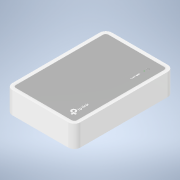
# Autodesk Inventor part: Network Switch (TL-SF1005D)
Saved by Autodesk Inventor 2020.1 (Build 241239000, 239)
## iProperties
Created: 2020-02-09
Part Number: Network Switch (TL-SF1005D)
Material: Generic
Document SubType Name: Modeling
Designer: tejas
Density: 1 g/cm^3
Appearance: Smooth - White
Author: tejas
Autodesk Inventor part; units mm, degrees
(part 1 of 2)
ref_plane "YZ Plane" through (0, 0, 0) normal (1, 0, 0) x (0, 1, 0)
ref_plane "XZ Plane" through (0, 0, 0) normal (0, 1, 0) x (-1, 0, 0)
ref_plane "XY Plane" through (0, 0, 0) normal (0, 0, 1) x (1, 0, 0)
sketch "Sketch1" plane through (0, 0, 0) normal (0, 1, 0) x (-1, 0, 0)
  line L0 (0, 0) -> (-71.12, 0)
  line L1 (-71.12, 0) -> (-71.12, -104.14)
  line L2 (-71.12, -104.14) -> (0, -104.14)
  line L3 (0, -104.14) -> (0, 0)
  dimension "d0" = 71.12
  dimension "d1" = 104.14
  constraints: 8 end point, 2 parallel, 1 horizontal, 1 perpendicular
  measures "d0" distance of L2.end L1.end
  measures "d1" distance of L1.end L0.end
extrude "Extrusion1" add sketch "Sketch1" along normal blind 22.86
sketch "Sketch2" plane through (0, 0, -104.14) normal (-1, 0, 0) x (0, 0, 1)
  line L0 (28.8163, 10.485) -> (16.9037, 10.485)
  line L1 (16.9037, 10.485) -> (16.9037, 12.4916)
  line L2 (16.9037, 12.4916) -> (16.51, 12.4916)
  line L3 (16.51, 12.4916) -> (16.51, 15.2856)
  line L4 (16.51, 15.2856) -> (16.9037, 15.2856)
  line L5 (16.9037, 15.2856) -> (16.9037, 17.3176)
  line L6 (16.9037, 17.3176) -> (19.7104, 17.3176)
  line L7 (19.7104, 17.3176) -> (19.7104, 18.222)
  line L8 (19.7104, 18.222) -> (20.828, 18.222)
  line L9 (20.828, 18.222) -> (20.828, 19.365)
  line L10 (20.828, 19.365) -> (24.892, 19.365)
  line L11 (22.86, 19.365) -> (22.86, 10.485) construction
  line L12 (28.8163, 10.485) -> (28.8163, 12.4916)
  line L13 (28.8163, 12.4916) -> (29.21, 12.4916)
  line L14 (29.21, 12.4916) -> (29.21, 15.2856)
  line L15 (29.21, 15.2856) -> (28.8163, 15.2856)
  line L16 (28.8163, 15.2856) -> (28.8163, 17.3176)
  line L17 (28.8163, 17.3176) -> (26.0096, 17.3176)
  line L18 (26.0096, 17.3176) -> (26.0096, 18.222)
  line L19 (26.0096, 18.222) -> (24.892, 18.222)
  line L20 (24.892, 18.222) -> (24.892, 19.365)
  line L21 (29.21, 13.8886) -> (30.48, 13.8886) construction
  line L22 (30.48, 13.8886) -> (30.48, 20.2386) construction
  line L23 (32.1437, 10.485) -> (44.0563, 10.485)
  line L24 (44.0563, 10.485) -> (44.0563, 12.4916)
  line L25 (44.0563, 12.4916) -> (44.45, 12.4916)
  line L26 (44.45, 12.4916) -> (44.45, 15.2856)
  line L27 (44.45, 15.2856) -> (44.0563, 15.2856)
  line L28 (44.0563, 15.2856) -> (44.0563, 17.3176)
  line L29 (44.0563, 17.3176) -> (41.2496, 17.3176)
  line L30 (41.2496, 17.3176) -> (41.2496, 18.222)
  line L31 (41.2496, 18.222) -> (40.132, 18.222)
  line L32 (40.132, 18.222) -> (40.132, 19.365)
  line L33 (40.132, 19.365) -> (36.068, 19.365)
  line L34 (38.1, 19.365) -> (38.1, 10.485) construction
  line L35 (36.068, 18.222) -> (36.068, 19.365)
  line L36 (34.9504, 18.222) -> (36.068, 18.222)
  line L37 (34.9504, 17.3176) -> (34.9504, 18.222)
  line L38 (32.1437, 17.3176) -> (34.9504, 17.3176)
  line L39 (32.1437, 15.2856) -> (32.1437, 17.3176)
  line L40 (31.75, 15.2856) -> (32.1437, 15.2856)
  line L41 (31.75, 12.4916) -> (31.75, 15.2856)
  line L42 (32.1437, 12.4916) -> (31.75, 12.4916)
  line L43 (32.1437, 10.485) -> (32.1437, 12.4916)
  line L44 (44.45, 13.8886) -> (45.085, 13.8886) construction
  line L45 (45.085, 13.8886) -> (45.085, 20.2386) construction
  line L46 (46.1137, 17.3176) -> (48.9204, 17.3176)
  line L47 (46.1137, 15.2856) -> (46.1137, 17.3176)
  line L48 (45.72, 15.2856) -> (46.1137, 15.2856)
  line L49 (46.1137, 12.4916) -> (45.72, 12.4916)
  line L50 (45.72, 12.4916) -> (45.72, 15.2856)
  line L51 (46.1137, 10.485) -> (46.1137, 12.4916)
  line L52 (58.0263, 10.485) -> (46.1137, 10.485)
  line L53 (55.2196, 17.3176) -> (55.2196, 18.222)
  line L54 (55.2196, 18.222) -> (54.102, 18.222)
  line L55 (48.9204, 17.3176) -> (48.9204, 18.222)
  line L56 (48.9204, 18.222) -> (50.038, 18.222)
  line L57 (54.102, 18.222) -> (54.102, 19.365)
  line L58 (50.038, 19.365) -> (54.102, 19.365)
  line L59 (50.038, 18.222) -> (50.038, 19.365)
  line L60 (52.07, 19.365) -> (52.07, 10.485) construction
  line L61 (58.0263, 17.3176) -> (55.2196, 17.3176)
  line L62 (58.0263, 15.2856) -> (58.0263, 17.3176)
  line L63 (58.42, 15.2856) -> (58.0263, 15.2856)
  line L64 (58.42, 12.4916) -> (58.42, 15.2856)
  line L65 (58.0263, 12.4916) -> (58.42, 12.4916)
  line L66 (58.0263, 10.485) -> (58.0263, 12.4916)
  line L67 (75.3237, 10.485) -> (87.2363, 10.485) construction
  line L68 (87.2363, 10.485) -> (87.2363, 12.4916) construction
  line L69 (87.2363, 12.4916) -> (87.63, 12.4916) construction
  line L70 (87.63, 12.4916) -> (87.63, 15.2856) construction
  line L71 (87.63, 15.2856) -> (87.2363, 15.2856) construction
  line L72 (87.2363, 15.2856) -> (87.2363, 17.3176) construction
  line L73 (87.2363, 17.3176) -> (84.4296, 17.3176) construction
  line L74 (84.4296, 17.3176) -> (84.4296, 18.222) construction
  line L75 (84.4296, 18.222) -> (83.312, 18.222) construction
  line L76 (83.312, 18.222) -> (83.312, 19.365) construction
  line L77 (83.312, 19.365) -> (79.248, 19.365) construction
  line L78 (81.28, 19.365) -> (81.28, 10.485) construction
  line L79 (79.248, 18.222) -> (79.248, 19.365) construction
  line L80 (78.1304, 18.222) -> (79.248, 18.222) construction
  line L81 (78.1304, 17.3176) -> (78.1304, 18.222) construction
  line L82 (75.3237, 17.3176) -> (78.1304, 17.3176) construction
  line L83 (75.3237, 15.2856) -> (75.3237, 17.3176) construction
  line L84 (74.93, 15.2856) -> (75.3237, 15.2856) construction
  line L85 (74.93, 12.4916) -> (74.93, 15.2856) construction
  line L86 (75.3237, 12.4916) -> (74.93, 12.4916) construction
  line L87 (75.3237, 10.485) -> (75.3237, 12.4916) construction
  line L88 (74.93, 13.8886) -> (73.66, 13.8886) construction
  line L89 (73.66, 13.8886) -> (73.66, 20.2386) construction
  line L90 (60.0837, 17.3176) -> (62.8904, 17.3176)
  line L91 (60.0837, 15.2856) -> (60.0837, 17.3176)
  line L92 (59.69, 15.2856) -> (60.0837, 15.2856)
  line L93 (60.0837, 12.4916) -> (59.69, 12.4916)
  line L94 (59.69, 12.4916) -> (59.69, 15.2856)
  line L95 (60.0837, 10.485) -> (60.0837, 12.4916)
  line L96 (71.9963, 10.485) -> (60.0837, 10.485)
  line L97 (69.1896, 17.3176) -> (69.1896, 18.222)
  line L98 (69.1896, 18.222) -> (68.072, 18.222)
  line L99 (62.8904, 17.3176) -> (62.8904, 18.222)
  line L100 (62.8904, 18.222) -> (64.008, 18.222)
  line L101 (68.072, 18.222) -> (68.072, 19.365)
  line L102 (64.008, 19.365) -> (68.072, 19.365)
  line L103 (64.008, 18.222) -> (64.008, 19.365)
  line L104 (66.04, 19.365) -> (66.04, 10.485) construction
  line L105 (71.9963, 17.3176) -> (69.1896, 17.3176)
  line L106 (71.9963, 15.2856) -> (71.9963, 17.3176)
  line L107 (72.39, 15.2856) -> (71.9963, 15.2856)
  line L108 (72.39, 12.4916) -> (72.39, 15.2856)
  line L109 (71.9963, 12.4916) -> (72.39, 12.4916)
  line L110 (71.9963, 10.485) -> (71.9963, 12.4916)
  line L111 (0, 0) -> (104.14, 0) construction
  line L112 (104.14, 0) -> (104.14, 22.86) construction
  line L113 (0, 22.86) -> (104.14, 22.86) construction
  line L114 (0, 0) -> (0, 22.86) construction
  line L115 (72.39, 13.8886) -> (73.025, 13.8886) construction
  line L116 (73.025, 13.8886) -> (73.025, 20.2386) construction
  line L117 (82.042, 19.365) -> (77.978, 19.365)
  line L118 (82.042, 18.222) -> (82.042, 19.365)
  line L119 (80.01, 19.365) -> (80.01, 10.485) construction
  line L120 (74.0537, 10.485) -> (85.9663, 10.485)
  line L121 (83.1596, 18.222) -> (82.042, 18.222)
  line L122 (83.1596, 17.3176) -> (83.1596, 18.222)
  line L123 (85.9663, 17.3176) -> (83.1596, 17.3176)
  line L124 (85.9663, 15.2856) -> (85.9663, 17.3176)
  line L125 (86.36, 15.2856) -> (85.9663, 15.2856)
  line L126 (85.9663, 10.485) -> (85.9663, 12.4916)
  line L127 (85.9663, 12.4916) -> (86.36, 12.4916)
  line L128 (86.36, 12.4916) -> (86.36, 15.2856)
  line L129 (73.66, 12.4916) -> (73.66, 15.2856)
  line L130 (73.66, 15.2856) -> (74.0537, 15.2856)
  line L131 (74.0537, 10.485) -> (74.0537, 12.4916)
  line L132 (74.0537, 12.4916) -> (73.66, 12.4916)
  line L133 (74.0537, 15.2856) -> (74.0537, 17.3176)
  line L134 (76.8604, 17.3176) -> (76.8604, 18.222)
  line L135 (74.0537, 17.3176) -> (76.8604, 17.3176)
  line L136 (77.978, 18.222) -> (77.978, 19.365)
  line L137 (76.8604, 18.222) -> (77.978, 18.222)
  point P0 (31.75, 13.8886)
  point P1 (58.42, 13.8886)
  point P2 (45.72, 13.8886)
  point P3 (59.69, 13.8886)
  point P4 (86.36, 13.8886)
  dimension "d4" = 11.9126
  dimension "d5" = 2.0066
  dimension "d6" = 0.3937
  dimension "d7" = 2.794
  dimension "d8" = 0.3937
  dimension "d9" = 2.032
  dimension "d10" = 2.8067
  dimension "d11" = 0.9044
  dimension "d12" = 1.1176
  dimension "d13" = 1.143
  dimension "d14" = 4.064
  dimension "d15" = 1.27
  dimension "d16" = 6.35
  dimension "d18" = 6.35
  dimension "d20" = 104.14
  dimension "d21" = 16.51
  dimension "d22" = 22.86
  dimension "d23" = 8.88
  dimension "d94" = 3.495
  dimension "d98" = 0.635
  dimension "d99" = 0.635
  constraints: 268 end point, 127 symmetric about line, 9 horizontal, 5 vertical, 4 midpoint, 3 perpendicular
  measures "d4" distance of L0.start L0.end
  measures "d5" distance of L0.end L1.end
  measures "d6" distance of L1.end L2.end
  measures "d7" distance of L2.end L3.end
  measures "d8" distance of L3.end L4.end
  measures "d9" distance of L4.end L5.end
  measures "d10" distance of L5.end L6.end
  measures "d11" distance of L6.end L7.end
  measures "d12" distance of L7.end L8.end
  measures "d13" distance of L8.end L9.end
  measures "d14" distance of L9.end L10.end
  measures "d15" distance of L21.start L21.end
  measures "d16" distance of L21.end L22.end
  measures "d18" distance of L44.end L45.end
  measures "d20" distance of L113.start L112.end
  measures "d21" distance from line of L114 L2.end
  measures "d22" distance of L111.start L113.start
  measures "d23" distance between parallel lines of L67 L77
  measures "d94" distance from line of L9.end L113
  measures "d98" distance of L44.start L44.end
  measures "d99" distance of L115.start L115.end
extrude "Extrusion2" cut sketch "Sketch2" against normal blind 11.2512
sketch "Sketch3" plane through (11.2512, 0, -104.14) normal (-1, 0, 0) x (0, 0, 1)
  line L0 (16.9037, 17.3176) -> (19.7104, 17.3176) construction
  line L1 (16.9037, 15.2856) -> (16.9037, 17.3176) construction
  line L2 (16.9037, 15.2856) -> (16.9037, 17.3176) construction
  line L3 (16.9037, 16.3016) -> (18.5417, 16.3016)
  line L4 (18.5417, 16.3016) -> (18.5417, 17.3176)
  line L5 (16.9037, 17.3176) -> (19.7104, 17.3176) construction
  line L6 (16.9037, 16.3016) -> (16.9037, 17.3176)
  line L7 (18.5417, 17.3176) -> (16.9037, 17.3176)
  line L8 (20.828, 19.365) -> (24.892, 19.365) construction
  line L9 (22.86, 19.365) -> (22.86, 10.485) construction
  line L10 (28.8163, 10.485) -> (16.9037, 10.485) construction
  line L11 (29.21, 15.2856) -> (29.21, 12.4916) construction
  line L12 (29.21, 13.8886) -> (29.845, 13.8886) construction
  line L13 (29.845, 13.8886) -> (29.845, 20.2386) construction
  line L14 (28.8163, 17.3176) -> (26.0096, 17.3176) construction
  line L15 (28.8163, 15.2856) -> (28.8163, 17.3176) construction
  line L16 (28.8163, 15.2856) -> (28.8163, 17.3176) construction
  line L17 (28.8163, 16.3016) -> (27.1783, 16.3016)
  line L18 (27.1783, 16.3016) -> (27.1783, 17.3176)
  line L19 (28.8163, 17.3176) -> (26.0096, 17.3176) construction
  line L20 (28.8163, 16.3016) -> (28.8163, 17.3176)
  line L21 (27.1783, 17.3176) -> (28.8163, 17.3176)
  line L22 (42.7863, 17.3176) -> (39.9796, 17.3176) construction
  line L23 (42.7863, 15.2856) -> (42.7863, 17.3176) construction
  line L24 (42.7863, 15.2856) -> (42.7863, 17.3176) construction
  line L25 (42.7863, 16.3016) -> (41.1483, 16.3016)
  line L26 (41.1483, 16.3016) -> (41.1483, 17.3176)
  line L27 (42.7863, 17.3176) -> (39.9796, 17.3176) construction
  line L28 (42.7863, 16.3016) -> (42.7863, 17.3176)
  line L29 (41.1483, 17.3176) -> (42.7863, 17.3176)
  line L30 (32.5117, 16.3016) -> (32.5117, 17.3176)
  line L31 (30.8737, 16.3016) -> (32.5117, 16.3016)
  line L32 (30.8737, 17.3176) -> (33.6804, 17.3176) construction
  line L33 (32.5117, 17.3176) -> (30.8737, 17.3176)
  line L34 (30.8737, 15.2856) -> (30.8737, 17.3176) construction
  line L35 (30.8737, 16.3016) -> (30.8737, 17.3176)
  line L36 (30.8737, 15.2856) -> (30.8737, 17.3176) construction
  line L37 (30.8737, 17.3176) -> (33.6804, 17.3176) construction
  line L38 (44.45, 15.2856) -> (44.45, 12.4916) construction
  line L39 (44.45, 13.8886) -> (45.085, 13.8886) construction
  line L40 (45.085, 13.8886) -> (45.085, 20.2386) construction
  line L41 (50.038, 19.365) -> (54.102, 19.365) construction
  line L42 (52.07, 19.365) -> (52.07, 6.99) construction
  line L43 (47.3837, 15.2856) -> (47.3837, 17.3176) construction
  line L44 (47.3837, 15.2856) -> (47.3837, 17.3176) construction
  line L45 (47.3837, 16.3016) -> (49.0217, 16.3016)
  line L46 (49.0217, 16.3016) -> (49.0217, 17.3176)
  line L47 (47.3837, 16.3016) -> (47.3837, 17.3176)
  line L48 (49.0217, 17.3176) -> (47.3837, 17.3176)
  line L49 (87.2363, 16.3016) -> (85.5983, 16.3016)
  line L50 (85.5983, 16.3016) -> (85.5983, 17.3176)
  line L51 (87.2363, 16.3016) -> (87.2363, 17.3176)
  line L52 (85.5983, 17.3176) -> (87.2363, 17.3176)
  line L53 (76.9617, 16.3016) -> (76.9617, 17.3176)
  line L54 (75.3237, 16.3016) -> (76.9617, 16.3016)
  line L55 (75.3237, 17.3176) -> (78.1304, 17.3176) construction
  line L56 (76.9617, 17.3176) -> (75.3237, 17.3176)
  line L57 (75.3237, 15.2856) -> (75.3237, 17.3176) construction
  line L58 (75.3237, 16.3016) -> (75.3237, 17.3176)
  line L59 (75.3237, 15.2856) -> (75.3237, 17.3176) construction
  line L60 (75.3237, 17.3176) -> (78.1304, 17.3176) construction
  line L61 (61.3537, 15.2856) -> (61.3537, 17.3176) construction
  line L62 (61.3537, 17.3176) -> (64.1604, 17.3176) construction
  line L63 (61.3537, 15.2856) -> (61.3537, 17.3176) construction
  line L64 (61.3537, 16.3016) -> (62.9917, 16.3016)
  line L65 (62.9917, 16.3016) -> (62.9917, 17.3176)
  line L66 (61.3537, 17.3176) -> (64.1604, 17.3176) construction
  line L67 (61.3537, 16.3016) -> (61.3537, 17.3176)
  line L68 (62.9917, 17.3176) -> (61.3537, 17.3176)
  line L69 (71.6283, 16.3016) -> (71.6283, 17.3176)
  line L70 (73.2663, 16.3016) -> (71.6283, 16.3016)
  line L71 (71.6283, 17.3176) -> (73.2663, 17.3176)
  line L72 (73.2663, 15.2856) -> (73.2663, 17.3176) construction
  line L73 (73.2663, 16.3016) -> (73.2663, 17.3176)
  line L74 (73.2663, 15.2856) -> (73.2663, 17.3176) construction
  line L75 (73.2663, 17.3176) -> (70.4596, 17.3176) construction
  line L76 (73.2663, 17.3176) -> (70.4596, 17.3176) construction
  line L77 (56.7563, 15.2856) -> (56.7563, 17.3176) construction
  line L78 (56.7563, 15.2856) -> (56.7563, 17.3176) construction
  line L79 (56.7563, 16.3016) -> (55.1183, 16.3016)
  line L80 (55.1183, 16.3016) -> (55.1183, 17.3176)
  line L81 (55.1183, 17.3176) -> (56.7563, 17.3176)
  line L82 (56.7563, 16.3016) -> (56.7563, 17.3176)
  line L83 (50.038, 18.222) -> (50.038, 19.365) construction
  point P0 (104.14, 0)
  point P1 (45.72, 15.2856)
  dimension "d27" = 1.638
  dimension "d28" = 0.635
  dimension "d29" = 6.35
  dimension "d31" = 0.635
  dimension "d32" = 6.35
  dimension "d33" = 4.064
  dimension "d34" = 2.032
  constraints: 148 end point, 51 symmetric about line, 7 point on line, 6 midpoint, 3 horizontal, 3 perpendicular, 2 collinear, 1 vertical
  measures "d27" distance of L3.start L3.end
  measures "d28" distance of L12.start L12.end
  measures "d29" distance of L12.end L13.end
  measures "d31" distance of L39.start L39.end
  measures "d32" distance of L39.end L40.end
  measures "d33" distance of L41.start L41.end
  measures "d34" distance between parallel lines of L42 L83
extrude "Extrusion3" add sketch "Sketch3" along normal blind 3.023
sketch "Sketch5" plane through (0, 10.485, -75.3237) normal (0, 1, 0) x (1, 0, 0)
  line L0 (4.6681, 8.4646) -> (3.7193, 8.4646)
  line L1 (3.7193, 8.4646) -> (3.7193, 7.9946)
  line L2 (3.7193, 7.9946) -> (4.6681, 7.9946)
  line L3 (4.6681, 7.9946) -> (4.6681, 8.4646)
  line L4 (4.1937, 7.9946) -> (4.1937, 7.7216) construction
  line L5 (4.1937, 7.7216) -> (3.4111, 7.7216) construction
  line L6 (4.1937, 8.4646) -> (4.1937, 8.7376) construction
  line L7 (4.1937, 8.7376) -> (3.4111, 8.7376) construction
  line L8 (4.6681, 6.9786) -> (3.7193, 6.9786)
  line L9 (3.7193, 6.9786) -> (3.7193, 7.4486)
  line L10 (3.7193, 7.4486) -> (4.6681, 7.4486)
  line L11 (4.6681, 7.4486) -> (4.6681, 6.9786)
  line L12 (4.1937, 7.4486) -> (4.1937, 7.7216) construction
  line L13 (4.1937, 6.9786) -> (4.1937, 6.7056) construction
  line L14 (4.1937, 6.7056) -> (3.4111, 6.7056) construction
  line L15 (4.6681, 4.9466) -> (3.7193, 4.9466)
  line L16 (3.7193, 4.9466) -> (3.7193, 5.4166)
  line L17 (3.7193, 5.4166) -> (4.6681, 5.4166)
  line L18 (4.6681, 5.4166) -> (4.6681, 4.9466)
  line L19 (4.1937, 5.4166) -> (4.1937, 5.6896) construction
  line L20 (4.1937, 5.6896) -> (3.4111, 5.6896) construction
  line L21 (4.1937, 4.9466) -> (4.1937, 4.6736) construction
  line L22 (4.1937, 4.6736) -> (3.4111, 4.6736) construction
  line L23 (4.1937, 5.9626) -> (4.1937, 5.6896) construction
  line L24 (3.7193, 5.9626) -> (4.6681, 5.9626)
  line L25 (4.6681, 5.9626) -> (4.6681, 6.4326)
  line L26 (4.6681, 6.4326) -> (3.7193, 6.4326)
  line L27 (3.7193, 6.4326) -> (3.7193, 5.9626)
  line L28 (4.1937, 6.4326) -> (4.1937, 6.7056) construction
  line L29 (4.6681, 0.8826) -> (3.7193, 0.8826)
  line L30 (3.7193, 0.8826) -> (3.7193, 1.3526)
  line L31 (3.7193, 1.3526) -> (4.6681, 1.3526)
  line L32 (4.6681, 1.3526) -> (4.6681, 0.8826)
  line L33 (4.1937, 1.3526) -> (4.1937, 1.6256) construction
  line L34 (4.1937, 1.6256) -> (3.4111, 1.6256) construction
  line L35 (4.1937, 0.8826) -> (4.1937, 0.6096) construction
  line L36 (4.1937, 0.6096) -> (3.4111, 0.6096) construction
  line L37 (4.1937, 1.8986) -> (4.1937, 1.6256) construction
  line L38 (3.7193, 1.8986) -> (4.6681, 1.8986)
  line L39 (4.6681, 1.8986) -> (4.6681, 2.3686)
  line L40 (4.6681, 2.3686) -> (3.7193, 2.3686)
  line L41 (3.7193, 2.3686) -> (3.7193, 1.8986)
  line L42 (4.1937, 2.3686) -> (4.1937, 2.6416) construction
  line L43 (4.1937, 2.6416) -> (3.4111, 2.6416) construction
  line L44 (4.6681, 2.9146) -> (3.7193, 2.9146)
  line L45 (4.1937, 2.9146) -> (4.1937, 2.6416) construction
  line L46 (4.6681, 3.3846) -> (4.6681, 2.9146)
  line L47 (3.7193, 3.3846) -> (4.6681, 3.3846)
  line L48 (3.7193, 2.9146) -> (3.7193, 3.3846)
  line L49 (4.1937, 3.3846) -> (4.1937, 3.6576) construction
  line L50 (4.1937, 3.6576) -> (3.4111, 3.6576) construction
  line L51 (4.1937, 3.9306) -> (4.1937, 3.6576) construction
  line L52 (3.7193, 3.9306) -> (4.6681, 3.9306)
  line L53 (4.6681, 3.9306) -> (4.6681, 4.4006)
  line L54 (3.7193, 4.4006) -> (3.7193, 3.9306)
  line L55 (4.6681, 4.4006) -> (3.7193, 4.4006)
  line L56 (4.1937, 4.4006) -> (4.1937, 4.6736) construction
  line L57 (3.7193, 0.8826) -> (3.7193, -2.3114) construction
  line L58 (3.7193, -2.3114) -> (3.4111, -2.3114) construction
  line L59 (4.6681, -13.0874) -> (3.7193, -13.0874)
  line L60 (3.7193, -13.0874) -> (3.7193, -12.6174)
  line L61 (3.7193, -12.6174) -> (4.6681, -12.6174)
  line L62 (4.6681, -12.6174) -> (4.6681, -13.0874)
  line L63 (4.1937, -12.6174) -> (4.1937, -12.3444) construction
  line L64 (4.1937, -12.3444) -> (3.4111, -12.3444) construction
  line L65 (4.1937, -13.0874) -> (4.1937, -13.3604) construction
  line L66 (4.1937, -13.3604) -> (3.4111, -13.3604) construction
  line L67 (4.1937, -12.0714) -> (4.1937, -12.3444) construction
  line L68 (3.7193, -12.0714) -> (4.6681, -12.0714)
  line L69 (4.6681, -12.0714) -> (4.6681, -11.6014)
  line L70 (4.6681, -11.6014) -> (3.7193, -11.6014)
  line L71 (3.7193, -11.6014) -> (3.7193, -12.0714)
  line L72 (4.1937, -11.6014) -> (4.1937, -11.3284) construction
  line L73 (4.1937, -11.3284) -> (3.4111, -11.3284) construction
  line L74 (4.6681, -11.0554) -> (3.7193, -11.0554)
  line L75 (4.1937, -11.0554) -> (4.1937, -11.3284) construction
  line L76 (4.6681, -10.5854) -> (4.6681, -11.0554)
  line L77 (3.7193, -10.5854) -> (4.6681, -10.5854)
  line L78 (3.7193, -11.0554) -> (3.7193, -10.5854)
  line L79 (4.1937, -10.5854) -> (4.1937, -10.3124) construction
  line L80 (4.1937, -10.3124) -> (3.4111, -10.3124) construction
  line L81 (4.1937, -10.0394) -> (4.1937, -10.3124) construction
  line L82 (3.7193, -10.0394) -> (4.6681, -10.0394)
  line L83 (4.6681, -10.0394) -> (4.6681, -9.5694)
  line L84 (3.7193, -9.5694) -> (3.7193, -10.0394)
  line L85 (4.6681, -9.5694) -> (3.7193, -9.5694)
  line L86 (4.1937, -9.5694) -> (4.1937, -9.2964) construction
  line L87 (4.1937, -9.2964) -> (3.4111, -9.2964) construction
  line L88 (4.6681, -6.9914) -> (3.7193, -6.9914)
  line L89 (4.1937, -6.9914) -> (4.1937, -7.2644) construction
  line L90 (4.1937, -7.2644) -> (3.4111, -7.2644) construction
  line L91 (4.1937, -7.5374) -> (4.1937, -7.2644) construction
  line L92 (4.6681, -7.5374) -> (3.7193, -7.5374)
  line L93 (4.6681, -8.0074) -> (4.6681, -7.5374)
  line L94 (3.7193, -8.0074) -> (4.6681, -8.0074)
  line L95 (3.7193, -7.5374) -> (3.7193, -8.0074)
  line L96 (4.1937, -8.0074) -> (4.1937, -8.2804) construction
  line L97 (4.1937, -8.2804) -> (3.4111, -8.2804) construction
  line L98 (4.1937, -8.5534) -> (4.1937, -8.2804) construction
  line L99 (3.7193, -8.5534) -> (4.6681, -8.5534)
  line L100 (3.7193, -9.0234) -> (3.7193, -8.5534)
  line L101 (4.6681, -8.5534) -> (4.6681, -9.0234)
  line L102 (4.6681, -9.0234) -> (3.7193, -9.0234)
  line L103 (4.1937, -9.0234) -> (4.1937, -9.2964) construction
  line L104 (4.6681, -5.5054) -> (3.7193, -5.5054)
  line L105 (3.7193, -5.5054) -> (3.7193, -5.9754)
  line L106 (3.7193, -5.9754) -> (4.6681, -5.9754)
  line L107 (4.6681, -5.9754) -> (4.6681, -5.5054)
  line L108 (4.1937, -5.9754) -> (4.1937, -6.2484) construction
  line L109 (4.6681, -6.5214) -> (4.6681, -6.9914)
  line L110 (3.7193, -6.9914) -> (3.7193, -6.5214)
  line L111 (3.7193, -6.5214) -> (4.6681, -6.5214)
  line L112 (4.1937, -6.2484) -> (3.4111, -6.2484) construction
  line L113 (4.1937, -5.5054) -> (4.1937, -5.2324) construction
  line L114 (4.1937, -5.2324) -> (3.4111, -5.2324) construction
  line L115 (4.1937, -6.5214) -> (4.1937, -6.2484) construction
  line L116 (3.7193, -5.5054) -> (3.7193, -2.3114) construction
  line L117 (3.7193, 8.4646) -> (3.7193, 11.6586) construction
  line L118 (3.7193, 11.6586) -> (3.4111, 11.6586) construction
  line L119 (3.7193, -13.0874) -> (3.7193, -16.2814) construction
  line L120 (3.7193, -16.2814) -> (3.4111, -16.2814) construction
  line L121 (4.6681, -41.0274) -> (3.7193, -41.0274)
  line L122 (3.7193, -41.0274) -> (3.7193, -40.5574)
  line L123 (3.7193, -40.5574) -> (4.6681, -40.5574)
  line L124 (4.6681, -40.5574) -> (4.6681, -41.0274)
  line L125 (4.1937, -40.5574) -> (4.1937, -40.2844) construction
  line L126 (4.1937, -40.2844) -> (3.4111, -40.2844) construction
  line L127 (4.1937, -41.0274) -> (4.1937, -41.3004) construction
  line L128 (4.1937, -41.3004) -> (3.4111, -41.3004) construction
  line L129 (4.1937, -40.0114) -> (4.1937, -40.2844) construction
  line L130 (3.7193, -40.0114) -> (4.6681, -40.0114)
  line L131 (4.6681, -40.0114) -> (4.6681, -39.5414)
  line L132 (4.6681, -39.5414) -> (3.7193, -39.5414)
  line L133 (3.7193, -39.5414) -> (3.7193, -40.0114)
  line L134 (4.1937, -39.5414) -> (4.1937, -39.2684) construction
  line L135 (4.1937, -39.2684) -> (3.4111, -39.2684) construction
  line L136 (4.6681, -38.9954) -> (3.7193, -38.9954)
  line L137 (4.1937, -38.9954) -> (4.1937, -39.2684) construction
  line L138 (4.6681, -38.5254) -> (4.6681, -38.9954)
  line L139 (3.7193, -38.5254) -> (4.6681, -38.5254)
  line L140 (3.7193, -38.9954) -> (3.7193, -38.5254)
  line L141 (4.1937, -38.5254) -> (4.1937, -38.2524) construction
  line L142 (4.1937, -38.2524) -> (3.4111, -38.2524) construction
  line L143 (4.1937, -37.9794) -> (4.1937, -38.2524) construction
  line L144 (3.7193, -37.9794) -> (4.6681, -37.9794)
  line L145 (4.6681, -37.9794) -> (4.6681, -37.5094)
  line L146 (3.7193, -37.5094) -> (3.7193, -37.9794)
  line L147 (4.6681, -37.5094) -> (3.7193, -37.5094)
  line L148 (4.1937, -37.5094) -> (4.1937, -37.2364) construction
  line L149 (4.1937, -37.2364) -> (3.4111, -37.2364) construction
  line L150 (4.6681, -34.9314) -> (3.7193, -34.9314)
  line L151 (4.1937, -34.9314) -> (4.1937, -35.2044) construction
  line L152 (4.1937, -35.2044) -> (3.4111, -35.2044) construction
  line L153 (4.1937, -35.4774) -> (4.1937, -35.2044) construction
  line L154 (4.6681, -35.4774) -> (3.7193, -35.4774)
  line L155 (4.6681, -35.9474) -> (4.6681, -35.4774)
  line L156 (3.7193, -35.9474) -> (4.6681, -35.9474)
  line L157 (3.7193, -35.4774) -> (3.7193, -35.9474)
  line L158 (4.1937, -35.9474) -> (4.1937, -36.2204) construction
  line L159 (4.1937, -36.2204) -> (3.4111, -36.2204) construction
  line L160 (4.1937, -36.4934) -> (4.1937, -36.2204) construction
  line L161 (3.7193, -36.4934) -> (4.6681, -36.4934)
  line L162 (3.7193, -36.9634) -> (3.7193, -36.4934)
  line L163 (4.6681, -36.4934) -> (4.6681, -36.9634)
  line L164 (4.6681, -36.9634) -> (3.7193, -36.9634)
  line L165 (4.1937, -36.9634) -> (4.1937, -37.2364) construction
  line L166 (4.6681, -33.4454) -> (3.7193, -33.4454)
  line L167 (3.7193, -33.4454) -> (3.7193, -33.9154)
  line L168 (3.7193, -33.9154) -> (4.6681, -33.9154)
  line L169 (4.6681, -33.9154) -> (4.6681, -33.4454)
  line L170 (4.1937, -33.9154) -> (4.1937, -34.1884) construction
  line L171 (4.6681, -34.4614) -> (4.6681, -34.9314)
  line L172 (3.7193, -34.9314) -> (3.7193, -34.4614)
  line L173 (3.7193, -34.4614) -> (4.6681, -34.4614)
  line L174 (4.1937, -34.1884) -> (3.4111, -34.1884) construction
  line L175 (4.1937, -33.4454) -> (4.1937, -33.1724) construction
  line L176 (4.1937, -33.1724) -> (3.4111, -33.1724) construction
  line L177 (4.1937, -34.4614) -> (4.1937, -34.1884) construction
  line L178 (3.7193, -33.4454) -> (3.7193, -30.2514) construction
  line L179 (3.7193, -30.2514) -> (3.4111, -30.2514) construction
  line L180 (3.7193, -20.4914) -> (4.6681, -20.4914)
  line L181 (4.6681, -20.4914) -> (4.6681, -20.9614)
  line L182 (4.6681, -20.9614) -> (3.7193, -20.9614)
  line L183 (4.1937, -20.9614) -> (4.1937, -21.2344) construction
  line L184 (4.1937, -21.2344) -> (3.4111, -21.2344) construction
  line L185 (4.1937, -21.5074) -> (4.1937, -21.2344) construction
  line L186 (4.6681, -21.5074) -> (3.7193, -21.5074)
  line L187 (4.6681, -21.9774) -> (4.6681, -21.5074)
  line L188 (3.7193, -21.9774) -> (4.6681, -21.9774)
  line L189 (4.1937, -22.2504) -> (3.4111, -22.2504) construction
  line L190 (4.1937, -21.9774) -> (4.1937, -22.2504) construction
  line L191 (4.1937, -22.5234) -> (4.1937, -22.2504) construction
  line L192 (3.7193, -22.5234) -> (4.6681, -22.5234)
  line L193 (4.6681, -22.5234) -> (4.6681, -22.9934)
  line L194 (4.6681, -22.9934) -> (3.7193, -22.9934)
  line L195 (4.1937, -23.2664) -> (3.4111, -23.2664) construction
  line L196 (4.1937, -23.5394) -> (4.1937, -23.2664) construction
  line L197 (4.6681, -23.5394) -> (3.7193, -23.5394)
  line L198 (3.7193, -24.0094) -> (4.6681, -24.0094)
  line L199 (4.6681, -24.0094) -> (4.6681, -23.5394)
  line L200 (4.1937, -24.0094) -> (4.1937, -24.2824) construction
  line L201 (4.1937, -22.9934) -> (4.1937, -23.2664) construction
  line L202 (4.1937, -24.2824) -> (3.4111, -24.2824) construction
  line L203 (4.1937, -24.5554) -> (4.1937, -24.2824) construction
  line L204 (3.7193, -24.5554) -> (4.6681, -24.5554)
  line L205 (4.6681, -24.5554) -> (4.6681, -25.0254)
  line L206 (4.6681, -25.0254) -> (3.7193, -25.0254)
  line L207 (4.1937, -25.2984) -> (3.4111, -25.2984) construction
  line L208 (4.1937, -25.0254) -> (4.1937, -25.2984) construction
  line L209 (4.6681, -25.5714) -> (3.7193, -25.5714)
  line L210 (4.1937, -25.5714) -> (4.1937, -25.2984) construction
  line L211 (4.6681, -26.0414) -> (4.6681, -25.5714)
  line L212 (3.7193, -26.0414) -> (4.6681, -26.0414)
  line L213 (4.1937, -26.0414) -> (4.1937, -26.3144) construction
  line L214 (4.1937, -26.3144) -> (3.4111, -26.3144) construction
  line L215 (4.1937, -26.5874) -> (4.1937, -26.3144) construction
  line L216 (3.7193, -26.5874) -> (4.6681, -26.5874)
  line L217 (4.6681, -19.4754) -> (3.7193, -19.4754)
  line L218 (4.1937, -20.4914) -> (4.1937, -20.2184) construction
  line L219 (4.1937, -20.2184) -> (3.4111, -20.2184) construction
  line L220 (4.1937, -19.9454) -> (4.1937, -20.2184) construction
  line L221 (3.7193, -19.9454) -> (4.6681, -19.9454)
  line L222 (4.1937, -19.4754) -> (4.1937, -19.2024) construction
  line L223 (4.1937, -19.2024) -> (3.4111, -19.2024) construction
  line L224 (4.6681, -19.9454) -> (4.6681, -19.4754)
  line L225 (4.6681, -26.5874) -> (4.6681, -27.0574)
  line L226 (4.6681, -27.0574) -> (3.7193, -27.0574)
  line L227 (4.1937, -27.0574) -> (4.1937, -27.3304) construction
  line L228 (4.1937, -27.3304) -> (3.4111, -27.3304) construction
  line L229 (3.7193, -21.5074) -> (3.7193, -21.9774)
  line L230 (3.7193, -22.9934) -> (3.7193, -22.5234)
  line L231 (3.7193, -23.5394) -> (3.7193, -24.0094)
  line L232 (3.7193, -19.4754) -> (3.7193, -19.9454)
  line L233 (3.7193, -20.9614) -> (3.7193, -20.4914)
  line L234 (3.7193, -25.5714) -> (3.7193, -26.0414)
  line L235 (3.7193, -25.0254) -> (3.7193, -24.5554)
  line L236 (3.7193, -27.0574) -> (3.7193, -26.5874)
  line L237 (3.7193, -27.0574) -> (3.7193, -30.2514) construction
  line L238 (3.7193, -41.0274) -> (3.7193, -44.2214) construction
  line L239 (3.7193, -44.2214) -> (3.4111, -44.2214) construction
  line L240 (3.7193, -19.4754) -> (3.7193, -16.2814) construction
  line L241 (4.1937, -48.4314) -> (4.1937, -48.1584) construction
  line L242 (4.1937, -48.1584) -> (3.4111, -48.1584) construction
  line L243 (4.1937, -47.8854) -> (4.1937, -48.1584) construction
  line L244 (3.7193, -47.8854) -> (4.6681, -47.8854)
  line L245 (4.6681, -47.4154) -> (3.7193, -47.4154)
  line L246 (4.6681, -47.8854) -> (4.6681, -47.4154)
  line L247 (3.7193, -47.4154) -> (3.7193, -47.8854)
  line L248 (3.7193, -48.4314) -> (4.6681, -48.4314)
  line L249 (4.6681, -48.4314) -> (4.6681, -48.9014)
  line L250 (3.7193, -48.9014) -> (3.7193, -48.4314)
  line L251 (4.6681, -48.9014) -> (3.7193, -48.9014)
  line L252 (4.1937, -48.9014) -> (4.1937, -49.1744) construction
  line L253 (4.1937, -49.1744) -> (3.4111, -49.1744) construction
  line L254 (4.1937, -49.4474) -> (4.1937, -49.1744) construction
  line L255 (4.6681, -49.4474) -> (3.7193, -49.4474)
  line L256 (4.6681, -49.9174) -> (4.6681, -49.4474)
  line L257 (3.7193, -49.4474) -> (3.7193, -49.9174)
  line L258 (3.7193, -49.9174) -> (4.6681, -49.9174)
  line L259 (4.1937, -49.9174) -> (4.1937, -50.1904) construction
  line L260 (4.1937, -50.1904) -> (3.4111, -50.1904) construction
  line L261 (4.1937, -50.4634) -> (4.1937, -50.1904) construction
  line L262 (3.7193, -50.4634) -> (4.6681, -50.4634)
  line L263 (4.6681, -50.4634) -> (4.6681, -50.9334)
  line L264 (3.7193, -50.9334) -> (3.7193, -50.4634)
  line L265 (4.6681, -50.9334) -> (3.7193, -50.9334)
  line L266 (4.1937, -50.9334) -> (4.1937, -51.2064) construction
  line L267 (4.1937, -51.2064) -> (3.4111, -51.2064) construction
  line L268 (4.1937, -51.4794) -> (4.1937, -51.2064) construction
  line L269 (4.6681, -51.4794) -> (3.7193, -51.4794)
  line L270 (3.7193, -51.4794) -> (3.7193, -51.9494)
  line L271 (4.6681, -51.9494) -> (4.6681, -51.4794)
  line L272 (4.1937, -51.9494) -> (4.1937, -52.2224) construction
  line L273 (3.7193, -51.9494) -> (4.6681, -51.9494)
  line L274 (4.1937, -52.4954) -> (4.1937, -52.2224) construction
  line L275 (3.7193, -52.4954) -> (4.6681, -52.4954)
  line L276 (4.6681, -52.4954) -> (4.6681, -52.9654)
  line L277 (4.6681, -52.9654) -> (3.7193, -52.9654)
  line L278 (3.7193, -52.9654) -> (3.7193, -52.4954)
  line L279 (4.1937, -53.2384) -> (3.4111, -53.2384) construction
  line L280 (4.1937, -52.9654) -> (4.1937, -53.2384) construction
  line L281 (4.1937, -52.2224) -> (3.4111, -52.2224) construction
  line L282 (4.6681, -53.5114) -> (3.7193, -53.5114)
  line L283 (4.1937, -53.5114) -> (4.1937, -53.2384) construction
  line L284 (4.6681, -53.9814) -> (4.6681, -53.5114)
  line L285 (3.7193, -53.5114) -> (3.7193, -53.9814)
  line L286 (3.7193, -53.9814) -> (4.6681, -53.9814)
  line L287 (4.1937, -53.9814) -> (4.1937, -54.2544) construction
  line L288 (4.1937, -54.2544) -> (3.4111, -54.2544) construction
  line L289 (4.1937, -54.5274) -> (4.1937, -54.2544) construction
  line L290 (4.6681, -54.5274) -> (4.6681, -54.9974)
  line L291 (3.7193, -54.9974) -> (3.7193, -54.5274)
  line L292 (4.6681, -54.9974) -> (3.7193, -54.9974)
  line L293 (3.7193, -54.5274) -> (4.6681, -54.5274)
  line L294 (4.1937, -54.9974) -> (4.1937, -55.2704) construction
  line L295 (4.1937, -55.2704) -> (3.4111, -55.2704) construction
  line L296 (3.7193, -54.9974) -> (3.7193, -58.1914) construction
  line L297 (4.1937, -47.4154) -> (4.1937, -47.1424) construction
  line L298 (4.1937, -47.1424) -> (3.4111, -47.1424) construction
  line L299 (3.7193, -47.4154) -> (3.7193, -44.2214) construction
  line L300 (0, 28.8163) -> (0, -75.3237) construction
  line L301 (71.12, 28.8163) -> (0, 28.8163) construction
  line L302 (3.7193, 8.4646) -> (4.1937, 8.4646) construction
  line L303 (4.1937, 8.4646) -> (4.1937, 8.2296) construction
  line L304 (4.1937, 8.2296) -> (3.7193, 8.2296) construction
  line L305 (3.7193, 8.2296) -> (3.7193, 8.4646) construction
  dimension "d37" = 0.47
  dimension "d38" = 0.9487
  dimension "d39" = 0.273
  dimension "d40" = 0.273
  dimension "d41" = 3.194
  dimension "d42" = 3.7193
  dimension "d43" = 20.3517
  dimension "d48" = 0.235
  dimension "d49" = 0.4744
  constraints: 608 end point, 329 symmetric about line, 4 horizontal, 4 parallel, 3 perpendicular, 3 vertical, 2 midpoint
  measures "d37" distance of L0.end L1.end
  measures "d38" distance of L1.end L2.end
  measures "d39" distance of L4.start L4.end
  measures "d40" distance of L6.start L6.end
  measures "d41" distance of L29.end L57.end
  measures "d42" distance from line of L300 L0.end
  measures "d43" distance from line of L301 L0.end
  measures "d48" distance of L302.end L303.end
  measures "d49" distance of L303.end L304.end
sketch "Sketch7" plane through (0, 10.485, -87.2363) normal (0, 0, 1) x (1, 0, 0)
  line L0 (11.2512, 0) -> (11.2512, 2.0066) projected
  line L1 (3.7193, 0) -> (11.2512, 2.8912)
  line L2 (3.7193, 0) -> (11.4459, 0) construction
  point P0 (0, -10.485)
  dimension "d50" = 21
  constraints: 4 end point, 1 horizontal, 1 point on line
  measures "d50" angle of L2 L1
sweep "Sweep1" add profiles "Sketch5" path "Sketch7" path curves L1 contours L27 L26 L25 L24 | L29 L30 L31 L32 | L41 L40 L39 L38 | L44 L48 L47 L46 | L59 L60 L61 L62 | L71 L70 L69 L68 | L74 L78 L77 L76 | L93 L94 L95 L92 | L121 L122 L123 L124 | L133 L132 L131 L130 | L136 L140 L139 L138 | L155 L156 L157 L154 | L187 L188 L229 L186 | L204 L205 L206 L235 | L211 L212 L234 L209 | L216 L225 L226 L236 | L256 L258 L257 L255 | L275 L276 L277 L278 | L284 L286 L285 L282 | L290 L292 L291 L293
sketch "Sketch8" plane through (0, 0, -104.14) normal (-1, 0, 0) x (0, 0, 1)
  circle A0 centre (74.0537, 18.222) radius 0.254
  circle A1 centre (60.0837, 18.222) radius 0.254
  circle A2 centre (46.1137, 18.222) radius 0.254
  circle A3 centre (32.1437, 18.222) radius 0.254
  circle A4 centre (16.9037, 18.222) radius 0.254
  line L0 (16.9037, 15.2856) -> (16.9037, 17.3176) projected
  line L1 (32.1437, 15.2856) -> (32.1437, 17.3176) projected
  line L2 (46.1137, 15.2856) -> (46.1137, 17.3176) projected
  line L3 (60.0837, 15.2856) -> (60.0837, 17.3176) projected
  line L4 (16.9037, 16.3016) -> (16.9037, 17.3176) projected
  line L5 (74.0537, 15.2856) -> (74.0537, 17.3176) projected
  line L6 (76.8604, 18.222) -> (77.978, 18.222) projected
  point P0 (104.14, 0)
  point P1 (16.9037, 16.8096)
  dimension "d53" = 0.508
  dimension "d54" = 0.508
  dimension "d55" = 0.508
  dimension "d56" = 0.508
  dimension "d57" = 0.508
  constraints: 5 centre point, 4 horizontal alignment, 1 midpoint, 1 point on line, 1 vertical alignment
  measures "d53" diameter of A0
  measures "d54" diameter of A1
  measures "d55" diameter of A2
  measures "d56" diameter of A3
  measures "d57" diameter of A4
extrude "Extrusion4" add sketch "Sketch8" along normal blind 0.127
fillet "Fillet1" radius 6.35 4 edges at (0, 11.43, 0) (71.12, 11.43, 0) (71.12, 11.43, -104.14) (0, 11.43, -104.14)